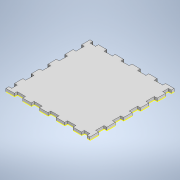
# Autodesk Inventor part: Lukt_botn
Saved by Autodesk Inventor 2021 (Build 250183000, 183)
## iProperties
Created: 2023-03-01
Part Number: Lukt_botn
Material: Generic
Document SubType Name: Modeling
Designer: frost
Density: 1 g/cm^3
Appearance: Default
Author: frost
Autodesk Inventor part; units mm, degrees
ref_plane "YZ Plane" through (0, 0, 0) normal (1, 0, 0) x (0, 1, 0)
ref_plane "XZ Plane" through (0, 0, 0) normal (0, 1, 0) x (-1, 0, 0)
ref_plane "XY Plane" through (0, 0, 0) normal (0, 0, 1) x (1, 0, 0)
sketch "Sketch1" plane through (0, 0, 0) normal (0, 1, 0) x (-1, 0, 0)
  line L0 (60, 60) -> (-60, 60)
  line L1 (-60, 60) -> (-60, -60)
  line L2 (-60, -60) -> (60, -60)
  line L3 (60, -60) -> (60, 60)
  point P0 (0, 0)
  dimension "d2" = 120
  dimension "d3" = 120
  dimension "d4" = 60
  dimension "d5" = 60
  constraints: 8 end point, 2 parallel, 1 horizontal, 1 perpendicular
  measures "d2" distance of L2.end L0.start
  measures "d3" distance of L1.end L2.end
  measures "d4" distance from line of L2 point (0, 0)
  measures "d5" distance from line of L3 point (0, 0)
extrude "Extrusion1" add sketch "Sketch1" along normal blind 4
sketch "Sketch2" plane through (-60, 0, -60) normal (-1, 0, 0) x (0, 0, 1)
  line L0 (12, 0) -> (24, 0)
  line L1 (24, 0) -> (24, 4)
  line L2 (24, 4) -> (12, 4)
  line L3 (12, 4) -> (12, 0)
  line L4 (0, 4) -> (120, 4) projected
  line L5 (0, 0) -> (0, 4) projected
  point P0 (60, 0)
  dimension "d8" = 12
  dimension "d9" = 4
  dimension "d10" = 0
  dimension "d11" = 12
  constraints: 8 end point, 2 parallel, 1 horizontal, 1 perpendicular
  measures "d8" distance of L1.end L2.end
  measures "d9" distance of L0.end L1.end
  measures "d10" distance between parallel lines of L4 L2
  measures "d11" distance between parallel lines of L5 L3
extrude "Extrusion2" cut sketch "Sketch2" against normal blind 4
pattern_linear "Rectangular Pattern1" count 5 spacing 24 along (0, 0, 1) of "Extrusion2"
sketch "Sketch3" plane through (-56, 0, 60) normal (-1, 0, 0) x (0, 0, 1)
  line L0 (0, 0) -> (-4, 0)
  line L1 (-4, 0) -> (-4, 4)
  line L2 (-4, 4) -> (0, 4)
  line L3 (0, 4) -> (0, 0)
  line L4 (0, 0) -> (0, 4) projected
  line L5 (0, 4) -> (-120, 4) projected
  point P0 (-60, 0)
  dimension "d23" = 4
  dimension "d24" = 4
  dimension "d25" = 0
  dimension "d26" = 0
  constraints: 8 end point, 2 parallel, 1 horizontal, 1 perpendicular
  measures "d23" distance of L0.end L1.end
  measures "d24" distance of L1.end L2.end
  measures "d25" distance between parallel lines of L4 L3
  measures "d26" distance between parallel lines of L5 L2
extrude "Extrusion3" add sketch "Sketch3" along normal blind 4
pattern_circular "Circular Pattern3" count 4 over 360 about axis through (0, -10, 0) along (0, 1, 0) of "Extrusion3", "Extrusion2", "Rectangular Pattern1"
sketch "Sketch4" plane through (0, 4, 0) normal (0, 1, 0) x (1, 0, 0)
  line L0 (-48, 56) -> (-56, 56) projected
  line L1 (-56, 56) -> (-56, 60) projected
  line L2 (-60, 60) -> (-56, 60) projected
  line L3 (-60, 60) -> (-60, 48) projected
  line L4 (-60, 48) -> (-56, 48) projected
  line L5 (-56, 48) -> (-56, 36) projected
  line L6 (-56, 36) -> (-60, 36) projected
  line L7 (-60, 36) -> (-60, 24) projected
  line L8 (-60, 24) -> (-56, 24) projected
  line L9 (-56, 24) -> (-56, 12) projected
  line L10 (-56, 12) -> (-60, 12) projected
  line L11 (-60, 12) -> (-60, 0) projected
  line L12 (-60, 0) -> (-56, 0) projected
  line L13 (-56, 0) -> (-56, -12) projected
  line L14 (-56, -12) -> (-60, -12) projected
  line L15 (-60, -12) -> (-60, -24) projected
  line L16 (-60, -24) -> (-56, -24) projected
  line L17 (-56, -24) -> (-56, -36) projected
  line L18 (-56, -36) -> (-60, -36) projected
  line L19 (-60, -36) -> (-60, -48) projected
  line L20 (-60, -48) -> (-56, -48) projected
  line L21 (-56, -48) -> (-56, -56) projected
  line L22 (-56, -56) -> (-60, -56) projected
  line L23 (-60, -60) -> (-60, -56) projected
  line L24 (-60, -60) -> (-48, -60) projected
  line L25 (-48, -60) -> (-48, -56) projected
  line L26 (-48, -56) -> (-36, -56) projected
  line L27 (-36, -56) -> (-36, -60) projected
  line L28 (-36, -60) -> (-24, -60) projected
  line L29 (-24, -60) -> (-24, -56) projected
  line L30 (-24, -56) -> (-12, -56) projected
  line L31 (-12, -56) -> (-12, -60) projected
  line L32 (-12, -60) -> (0, -60) projected
  line L33 (0, -60) -> (0, -56) projected
  line L34 (0, -56) -> (12, -56) projected
  line L35 (12, -56) -> (12, -60) projected
  line L36 (12, -60) -> (24, -60) projected
  line L37 (24, -60) -> (24, -56) projected
  line L38 (24, -56) -> (36, -56) projected
  line L39 (36, -56) -> (36, -60) projected
  line L40 (36, -60) -> (48, -60) projected
  line L41 (48, -60) -> (48, -56) projected
  line L42 (48, -56) -> (56, -56) projected
  line L43 (56, -56) -> (56, -60) projected
  line L44 (60, -60) -> (56, -60) projected
  line L45 (60, -60) -> (60, -48) projected
  line L46 (60, -48) -> (56, -48) projected
  line L47 (56, -48) -> (56, -36) projected
  line L48 (56, -36) -> (60, -36) projected
  line L49 (60, -36) -> (60, -24) projected
  line L50 (60, -24) -> (56, -24) projected
  line L51 (56, -24) -> (56, -12) projected
  line L52 (56, -12) -> (60, -12) projected
  line L53 (60, -12) -> (60, 0) projected
  line L54 (60, 0) -> (56, 0) projected
  line L55 (56, 0) -> (56, 12) projected
  line L56 (56, 12) -> (60, 12) projected
  line L57 (60, 12) -> (60, 24) projected
  line L58 (60, 24) -> (56, 24) projected
  line L59 (56, 24) -> (56, 36) projected
  line L60 (56, 36) -> (60, 36) projected
  line L61 (60, 36) -> (60, 48) projected
  line L62 (60, 48) -> (56, 48) projected
  line L63 (56, 48) -> (56, 56) projected
  line L64 (56, 56) -> (60, 56) projected
  line L65 (60, 60) -> (60, 56) projected
  line L66 (60, 60) -> (48, 60) projected
  line L67 (48, 60) -> (48, 56) projected
  line L68 (48, 56) -> (36, 56) projected
  line L69 (36, 56) -> (36, 60) projected
  line L70 (36, 60) -> (24, 60) projected
  line L71 (24, 60) -> (24, 56) projected
  line L72 (24, 56) -> (12, 56) projected
  line L73 (12, 56) -> (12, 60) projected
  line L74 (12, 60) -> (0, 60) projected
  line L75 (0, 60) -> (0, 56) projected
  line L76 (0, 56) -> (-12, 56) projected
  line L77 (-12, 56) -> (-12, 60) projected
  line L78 (-12, 60) -> (-24, 60) projected
  line L79 (-24, 60) -> (-24, 56) projected
  line L80 (-24, 56) -> (-36, 56) projected
  line L81 (-36, 56) -> (-36, 60) projected
  line L82 (-36, 60) -> (-48, 60) projected
  line L83 (-48, 60) -> (-48, 56) projected
  line L84 (-48.11, 60.11) -> (-35.89, 60.11)
  line L85 (-35.89, 60.11) -> (-35.89, 56.11)
  line L86 (-35.89, 56.11) -> (-24.11, 56.11)
  line L87 (-24.11, 56.11) -> (-24.11, 60.11)
  line L88 (-24.11, 60.11) -> (-11.89, 60.11)
  line L89 (-11.89, 60.11) -> (-11.89, 56.11)
  line L90 (-11.89, 56.11) -> (-0.11, 56.11)
  line L91 (-0.11, 56.11) -> (-0.11, 60.11)
  line L92 (-0.11, 60.11) -> (12.11, 60.11)
  line L93 (12.11, 60.11) -> (12.11, 56.11)
  line L94 (12.11, 56.11) -> (23.89, 56.11)
  line L95 (23.89, 56.11) -> (23.89, 60.11)
  line L96 (23.89, 60.11) -> (36.11, 60.11)
  line L97 (36.11, 60.11) -> (36.11, 56.11)
  line L98 (36.11, 56.11) -> (47.89, 56.11)
  line L99 (47.89, 56.11) -> (47.89, 60.11)
  line L100 (47.89, 60.11) -> (60.11, 60.11)
  line L101 (60.11, 60.11) -> (60.11, 55.89)
  line L102 (60.11, 55.89) -> (56.11, 55.89)
  line L103 (56.11, 55.89) -> (56.11, 48.11)
  line L104 (56.11, 48.11) -> (60.11, 48.11)
  line L105 (60.11, 48.11) -> (60.11, 35.89)
  line L106 (60.11, 35.89) -> (56.11, 35.89)
  line L107 (56.11, 35.89) -> (56.11, 24.11)
  line L108 (56.11, 24.11) -> (60.11, 24.11)
  line L109 (60.11, 24.11) -> (60.11, 11.89)
  line L110 (60.11, 11.89) -> (56.11, 11.89)
  line L111 (56.11, 11.89) -> (56.11, 0.11)
  line L112 (56.11, 0.11) -> (60.11, 0.11)
  line L113 (60.11, 0.11) -> (60.11, -12.11)
  line L114 (60.11, -12.11) -> (56.11, -12.11)
  line L115 (56.11, -12.11) -> (56.11, -23.89)
  line L116 (56.11, -23.89) -> (60.11, -23.89)
  line L117 (60.11, -23.89) -> (60.11, -36.11)
  line L118 (60.11, -36.11) -> (56.11, -36.11)
  line L119 (56.11, -36.11) -> (56.11, -47.89)
  line L120 (56.11, -47.89) -> (60.11, -47.89)
  line L121 (60.11, -47.89) -> (60.11, -60.11)
  line L122 (60.11, -60.11) -> (55.89, -60.11)
  line L123 (55.89, -60.11) -> (55.89, -56.11)
  line L124 (55.89, -56.11) -> (48.11, -56.11)
  line L125 (48.11, -56.11) -> (48.11, -60.11)
  line L126 (48.11, -60.11) -> (35.89, -60.11)
  line L127 (35.89, -60.11) -> (35.89, -56.11)
  line L128 (35.89, -56.11) -> (24.11, -56.11)
  line L129 (24.11, -56.11) -> (24.11, -60.11)
  line L130 (24.11, -60.11) -> (11.89, -60.11)
  line L131 (11.89, -60.11) -> (11.89, -56.11)
  line L132 (11.89, -56.11) -> (0.11, -56.11)
  line L133 (0.11, -56.11) -> (0.11, -60.11)
  line L134 (0.11, -60.11) -> (-12.11, -60.11)
  line L135 (-12.11, -60.11) -> (-12.11, -56.11)
  line L136 (-12.11, -56.11) -> (-23.89, -56.11)
  line L137 (-23.89, -56.11) -> (-23.89, -60.11)
  line L138 (-23.89, -60.11) -> (-36.11, -60.11)
  line L139 (-36.11, -60.11) -> (-36.11, -56.11)
  line L140 (-36.11, -56.11) -> (-47.89, -56.11)
  line L141 (-47.89, -56.11) -> (-47.89, -60.11)
  line L142 (-47.89, -60.11) -> (-60.11, -60.11)
  line L143 (-60.11, -60.11) -> (-60.11, -55.89)
  line L144 (-60.11, -55.89) -> (-56.11, -55.89)
  line L145 (-56.11, -55.89) -> (-56.11, -48.11)
  line L146 (-56.11, -48.11) -> (-60.11, -48.11)
  line L147 (-60.11, -48.11) -> (-60.11, -35.89)
  line L148 (-60.11, -35.89) -> (-56.11, -35.89)
  line L149 (-56.11, -35.89) -> (-56.11, -24.11)
  line L150 (-56.11, -24.11) -> (-60.11, -24.11)
  line L151 (-60.11, -24.11) -> (-60.11, -11.89)
  line L152 (-60.11, -11.89) -> (-56.11, -11.89)
  line L153 (-56.11, -11.89) -> (-56.11, -0.11)
  line L154 (-56.11, -0.11) -> (-60.11, -0.11)
  line L155 (-60.11, -0.11) -> (-60.11, 12.11)
  line L156 (-60.11, 12.11) -> (-56.11, 12.11)
  line L157 (-56.11, 12.11) -> (-56.11, 23.89)
  line L158 (-56.11, 23.89) -> (-60.11, 23.89)
  line L159 (-60.11, 23.89) -> (-60.11, 36.11)
  line L160 (-60.11, 36.11) -> (-56.11, 36.11)
  line L161 (-56.11, 36.11) -> (-56.11, 47.89)
  line L162 (-56.11, 47.89) -> (-60.11, 47.89)
  line L163 (-60.11, 47.89) -> (-60.11, 60.11)
  line L164 (-60.11, 60.11) -> (-55.89, 60.11)
  line L165 (-55.89, 60.11) -> (-55.89, 56.11)
  line L166 (-55.89, 56.11) -> (-48.11, 56.11)
  line L167 (-48.11, 56.11) -> (-48.11, 60.11)
  point P0 (0, 0)
  dimension "d32" = 0.11
  constraints: 168 end point, 83 other
  measures "d32" distance between parallel lines of L82 L84
extrude "Extrusion4" add sketch "Sketch4" against normal blind 4 contours L83 L82 L81 L80 L79 L78 L77 L76 L75 L74 L73 L72 L71 L70 L69 L68 L67 L66 L65 L64 L63 L62 L61 L60 L59 L58 L57 L56 L55 L54 L53 L52 L51 L50 L49 L48 L47 L46 L45 L44 L43 L42 L41 L40 L39 L38 L37 L36 L35 L34 L33 L32 L31 L30 L29 L28 L27 L26 L25 L24 L23 L22 L21 L20 L19 L18 L17 L16 L15 L14 L13 L12 L11 L10 L9 L8 L7 L6 L5 L4 L3 L2 L1 L0 | L84 L85 L86 L87 L88 L89 L90 L91 L92 L93 L94 L95 L96 L97 L98 L99 L100 L101 L102 L103 L104 L105 L106 L107 L108 L109 L110 L111 L112 L113 L114 L115 L116 L117 L118 L119 L120 L121 L122 L123 L124 L125 L126 L127 L128 L129 L130 L131 L132 L133 L134 L135 L136 L137 L138 L139 L140 L141 L142 L143 L144 L145 L146 L147 L148 L149 L150 L151 L152 L153 L154 L155 L156 L157 L158 L159 L160 L161 L162 L163 L164 L165 L166 L167
sketch "Sketch5" plane through (0, 0, 0) normal (0, -1, 0) x (1, 0, 0)
  line L0 (-55.89, -56.11) -> (-48.11, -56.11) projected
  line L1 (-48.11, -56.11) -> (-48.11, -60.11) projected
  line L2 (-48.11, -60.11) -> (-35.89, -60.11) projected
  line L3 (-35.89, -60.11) -> (-35.89, -56.11) projected
  line L4 (-35.89, -56.11) -> (-24.11, -56.11) projected
  line L5 (-24.11, -56.11) -> (-24.11, -60.11) projected
  line L6 (-24.11, -60.11) -> (-11.89, -60.11) projected
  line L7 (-11.89, -60.11) -> (-11.89, -56.11) projected
  line L8 (-11.89, -56.11) -> (-0.11, -56.11) projected
  line L9 (-0.11, -56.11) -> (-0.11, -60.11) projected
  line L10 (-0.11, -60.11) -> (12.11, -60.11) projected
  line L11 (12.11, -60.11) -> (12.11, -56.11) projected
  line L12 (12.11, -56.11) -> (23.89, -56.11) projected
  line L13 (23.89, -56.11) -> (23.89, -60.11) projected
  line L14 (23.89, -60.11) -> (36.11, -60.11) projected
  line L15 (36.11, -60.11) -> (36.11, -56.11) projected
  line L16 (36.11, -56.11) -> (47.89, -56.11) projected
  line L17 (47.89, -56.11) -> (47.89, -60.11) projected
  line L18 (47.89, -60.11) -> (60.11, -60.11) projected
  line L19 (60.11, -60.11) -> (60.11, -55.89) projected
  line L20 (60.11, -55.89) -> (56.11, -55.89) projected
  line L21 (56.11, -55.89) -> (56.11, -48.11) projected
  line L22 (56.11, -48.11) -> (60.11, -48.11) projected
  line L23 (60.11, -48.11) -> (60.11, -35.89) projected
  line L24 (60.11, -35.89) -> (56.11, -35.89) projected
  line L25 (56.11, -35.89) -> (56.11, -24.11) projected
  line L26 (56.11, -24.11) -> (60.11, -24.11) projected
  line L27 (60.11, -24.11) -> (60.11, -11.89) projected
  line L28 (60.11, -11.89) -> (56.11, -11.89) projected
  line L29 (56.11, -11.89) -> (56.11, -0.11) projected
  line L30 (56.11, -0.11) -> (60.11, -0.11) projected
  line L31 (60.11, -0.11) -> (60.11, 12.11) projected
  line L32 (60.11, 12.11) -> (56.11, 12.11) projected
  line L33 (56.11, 12.11) -> (56.11, 23.89) projected
  line L34 (56.11, 23.89) -> (60.11, 23.89) projected
  line L35 (60.11, 23.89) -> (60.11, 36.11) projected
  line L36 (60.11, 36.11) -> (56.11, 36.11) projected
  line L37 (56.11, 36.11) -> (56.11, 47.89) projected
  line L38 (56.11, 47.89) -> (60.11, 47.89) projected
  line L39 (60.11, 47.89) -> (60.11, 60.11) projected
  line L40 (60.11, 60.11) -> (55.89, 60.11) projected
  line L41 (55.89, 60.11) -> (55.89, 56.11) projected
  line L42 (55.89, 56.11) -> (48.11, 56.11) projected
  line L43 (48.11, 56.11) -> (48.11, 60.11) projected
  line L44 (48.11, 60.11) -> (35.89, 60.11) projected
  line L45 (35.89, 60.11) -> (35.89, 56.11) projected
  line L46 (35.89, 56.11) -> (24.11, 56.11) projected
  line L47 (24.11, 56.11) -> (24.11, 60.11) projected
  line L48 (24.11, 60.11) -> (11.89, 60.11) projected
  line L49 (11.89, 60.11) -> (11.89, 56.11) projected
  line L50 (11.89, 56.11) -> (0.11, 56.11) projected
  line L51 (0.11, 56.11) -> (0.11, 60.11) projected
  line L52 (0.11, 60.11) -> (-12.11, 60.11) projected
  line L53 (-12.11, 60.11) -> (-12.11, 56.11) projected
  line L54 (-12.11, 56.11) -> (-23.89, 56.11) projected
  line L55 (-23.89, 56.11) -> (-23.89, 60.11) projected
  line L56 (-23.89, 60.11) -> (-36.11, 60.11) projected
  line L57 (-36.11, 60.11) -> (-36.11, 56.11) projected
  line L58 (-36.11, 56.11) -> (-47.89, 56.11) projected
  line L59 (-47.89, 56.11) -> (-47.89, 60.11) projected
  line L60 (-47.89, 60.11) -> (-60.11, 60.11) projected
  line L61 (-60.11, 60.11) -> (-60.11, 55.89) projected
  line L62 (-60.11, 55.89) -> (-56.11, 55.89) projected
  line L63 (-56.11, 55.89) -> (-56.11, 48.11) projected
  line L64 (-56.11, 48.11) -> (-60.11, 48.11) projected
  line L65 (-60.11, 48.11) -> (-60.11, 35.89) projected
  line L66 (-60.11, 35.89) -> (-56.11, 35.89) projected
  line L67 (-56.11, 35.89) -> (-56.11, 24.11) projected
  line L68 (-56.11, 24.11) -> (-60.11, 24.11) projected
  line L69 (-60.11, 24.11) -> (-60.11, 11.89) projected
  line L70 (-60.11, 11.89) -> (-56.11, 11.89) projected
  line L71 (-56.11, 11.89) -> (-56.11, 0.11) projected
  line L72 (-56.11, 0.11) -> (-60.11, 0.11) projected
  line L73 (-60.11, 0.11) -> (-60.11, -12.11) projected
  line L74 (-60.11, -12.11) -> (-56.11, -12.11) projected
  line L75 (-56.11, -12.11) -> (-56.11, -23.89) projected
  line L76 (-56.11, -23.89) -> (-60.11, -23.89) projected
  line L77 (-60.11, -23.89) -> (-60.11, -36.11) projected
  line L78 (-60.11, -36.11) -> (-56.11, -36.11) projected
  line L79 (-56.11, -36.11) -> (-56.11, -47.89) projected
  line L80 (-56.11, -47.89) -> (-60.11, -47.89) projected
  line L81 (-60.11, -47.89) -> (-60.11, -60.11) projected
  line L82 (-60.11, -60.11) -> (-55.89, -60.11) projected
  line L83 (-55.89, -60.11) -> (-55.89, -56.11) projected
  point P0 (0, 0)
equation "\"d2\" = width"
equation "\"d3\" = height"
equation "\"d4\" = 0.5 * width"
equation "\"d5\" = 0.5 * height"
equation "\"d8\" = finger"
equation "\"d9\" = thickness"
equation "\"d11\" = finger"
equation "\"d19\" = 2 * finger"
equation "\"d23\" = thickness"
equation "\"d24\" = 0.333333 * finger"
equation "\"d27\" = thickness"
equation "\"d32\" = 0.5 * kerf"
equation "\"d33\" = thickness"
equation "\"width\" = 120"
equation "\"height\" = 120"
equation "\"finger\" = 12"
equation "\"thickness\" = 4"
equation "\"kerf\" = 0.22"
body "Solid1"
